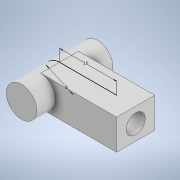
# Autodesk Inventor part: Pitch and Yaw
Saved by Autodesk Inventor 2020 (Build 240168000, 168)
## iProperties
Created: 2020-12-23
Part Number: Pitch and Yaw
Material: Generic
Document SubType Name: Modeling
Designer: frost
Density: 1 g/cm^3
Appearance: Default
Author: frost
Autodesk Inventor part; units mm, degrees
ref_plane "YZ Plane" through (0, 0, 0) normal (1, 0, 0) x (0, 1, 0)
ref_plane "XZ Plane" through (0, 0, 0) normal (0, 1, 0) x (-1, 0, 0)
ref_plane "XY Plane" through (0, 0, 0) normal (0, 0, 1) x (1, 0, 0)
sketch "Sketch1" plane through (0, 0, 0) normal (0, 0, 1) x (1, 0, 0)
  circle A0 centre (0, 0) radius 4
  line L0 (15, 1) -> (15, 4)
  line L1 (4, 0) -> (7.8423, 0)
  line L2 (15, 4) -> (0, 4)
  line L3 (15, -1) -> (15, -4)
  line L4 (15, -4) -> (0, -4)
  line L5 (15, 1) -> (15, -1)
  point P0 (0, -4)
  dimension "d0" = 8
  dimension "d2" = 15
  constraints: 12 end point, 3 symmetric about line, 2 point on circle, 2 vertical, 1 centre point, 1 coincident, 1 horizontal, 1 parallel, 1 tangent
  measures "d0" diameter of A0
  measures "d2" distance of L0.end L2.end
extrude "Extrusion1" add sketch "Sketch1" along normal mid plane 10 contours A0 L2 L0 L5 L3 L4
extrude "Extrusion2" add sketch "Sketch1" along normal mid plane 20 contours A0
sketch "Sketch2" plane through (15, -4, 5) normal (1, 0, 0) x (0, 0, -1)
  circle A0 centre (5, 4) radius 2.5
  line L0 (0, 0) -> (0, 8) projected
  line L1 (10, 8) -> (10, 0) projected
  line L2 (0, 8) -> (10, 8)
  line L3 (10, 8) -> (10, 0)
  line L4 (10, 0) -> (0, 0)
  line L5 (0, 0) -> (0, 8)
  dimension "d7" = 5
  constraints: 8 end point, 2 parallel, 1 centre point, 1 coincident, 1 horizontal, 1 perpendicular
  measures "d7" diameter of A0
extrude "Extrusion3" add sketch "Sketch2" along normal blind 5
body "Solid1"
